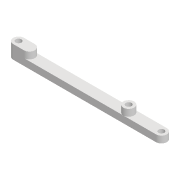
# Autodesk Inventor part: Part_2
Saved by Autodesk Inventor 2022 (Build 260153000, 153)
## iProperties
Created: 2022-04-21
Part Number: Part_2
Material: Generic
Document SubType Name: Modeling
Designer: dell
Density: 1 g/cm^3
Appearance: Default
Author: dell
Autodesk Inventor part; units mm, degrees
ref_plane "YZ Plane" through (0, 0, 0) normal (1, 0, 0) x (0, 1, 0)
ref_plane "XZ Plane" through (0, 0, 0) normal (0, 1, 0) x (-1, 0, 0)
ref_plane "XY Plane" through (0, 0, 0) normal (0, 0, 1) x (1, 0, 0)
sketch "Sketch1" plane through (0, 0, 0) normal (0, 1, 0) x (-1, 0, 0)
  line L0 (0, 0) -> (-105.445, 0) construction
  line L1 (0, 4) -> (-105.445, 4)
  line L2 (-105.445, -4) -> (0, -4)
  arc A0 (0, -4) -> (0, 4) centre (0, 0) ccw
  arc A1 (-105.445, 4) -> (-105.445, -4) centre (-105.445, 0) ccw
  circle A2 centre (0, 0) radius 2.1
  circle A3 centre (-81.271, 0) radius 2.1
  circle A4 centre (-105.445, 0) radius 2.1
  point P0 (-52.7225, 0)
  point P1 (-52.7225, 0)
  dimension "d0" = 105.445
  dimension "d1" = 8
  dimension "d2" = 4.2
  dimension "d8" = 4.2
  dimension "d9" = 81.271
  dimension "d10" = 4.2
  constraints: 8 end point, 5 centre point, 4 point on circle, 4 tangent, 2 coincident, 1 horizontal, 1 midpoint, 1 parallel, 1 point on line
  measures "d0" distance of L0.end L0.start
  measures "d1" distance between parallel lines of L1 L2
  measures "d2" diameter of A2
  measures "d8" diameter of A3
  measures "d9" distance of L0.start A3.centre
  measures "d10" diameter of A4
extrude "Extrusion1" add sketch "Sketch1" along normal blind 5
sketch "Sketch2" plane through (0, 5, 0) normal (0, 1, 0) x (1, 0, 0)
  arc A0 (105.445, -4) -> (105.445, 4) centre (105.445, 0) ccw projected
  line L0 (105.445, 4) -> (0, 4) projected
  arc A1 (0, 4) -> (0, -4) centre (0, 0) ccw projected
  line L1 (0, -4) -> (105.445, -4) projected
  circle A2 centre (81.271, 0) radius 2.1 projected
  circle A3 centre (105.445, 0) radius 2.1 projected
  circle A4 centre (0, 0) radius 2.1 projected
  circle A5 centre (8, 0) radius 4
  line L2 (0, -4) -> (105.445, -4) projected
  circle A6 centre (97.445, 0) radius 4
  circle A7 centre (81.271, 0) radius 4
  point P0 (97.445, -4)
  point P1 (97.445, 4)
  point P2 (8, -4)
  point P3 (8, 4)
  dimension "d11" = 8
  dimension "d12" = 8
  dimension "d13" = 8
  dimension "d28" = 8
  constraints: 3 centre point, 1 coincident, 1 tangent
  measures "d11" distance of point (0, 0) A5.centre
  measures "d12" diameter of A6
  measures "d13" distance of A0.centre A6.centre
  measures "d28" diameter of A7
extrude "Extrusion7" add sketch "Sketch2" along normal blind 5 contours A7 | L1 A1 L0 A5 | A5
body "Solid1"
